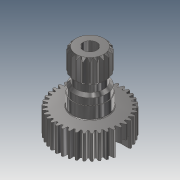
# Autodesk Inventor part: Цилиндрическое зубчатое зацепление2
Saved by Autodesk Inventor 2017 (Build 210142000, 142)
## iProperties
Created: 2018-08-24
Part Number: Цилиндрическое зубчатое зацепление2
Material: Сталь нержавеющая, 440C
Document SubType Name: Modeling
Designer: Shepelev
Categories: <?xml version="1.0" encoding="UTF-16"?> <MemberInstance><Categories><FamilyTemplate><FamilyTemplateParameter ValueType="xs:double" Id="1" ObjectReferenceKey="da_z" ObjectType="kUserParameterObject"/><FamilyTemplateParameter ValueType="xs:double" Id="2" ObjectReferenceKey="da_b" ObjectType="kUserParameterObject"/><FamilyTemplateParameter ValueType="xs:double" Id="3" ObjectReferenceKey="da_beta" ObjectType="kUserParameterObject"/><FamilyTemplateParameter ValueType="xs:double" Id="4" ObjectReferenceKey="da_da" ObjectType="kUserParameterObject"/><FamilyTemplateParameter ValueType="xs:double" Id="5" ObjectReferenceKey="da_aw" ObjectType="kUserParameterObject"/><FamilyTemplateParameter ValueType="xs:string" Id="6" ObjectReferenceKey="EAIAABAAAACIAQAAAAAAAIAAAAAAAAAA" ObjectType="83910656" SubObjectId="SurfaceGeometry"/></FamilyTemplate><ParamToTemplateMap><ParamToTemplate CategoryParameter="//CategoryParameter[@InternalName='046C89C9-8512-4d59-83FE-43B91F4F132A']" TemplateParameter="1"/><ParamToTemplate CategoryParameter="//CategoryParameter[@InternalName='2552DF32-E462-4b46-AEBF-C6C7768E72AC']" TemplateParameter="2"/><ParamToTemplate CategoryParameter="//CategoryParameter[@InternalName='C9EE641D-15FC-4fae-A226-E94C4372FDD7']" TemplateParameter="3"/><ParamToTemplate><ParamToTemplate CategoryParameter="//CategoryParameter[@InternalName='00B6519A-459B-49c7-AD84-2E56D39A5744']" ConstantValue="-0.270000"/></ParamToTemplate><ParamToTemplate><ParamToTemplate CategoryParameter="//CategoryParameter[@InternalName='04B31F0E-C7A6-4894-AA32-9629BEFACF47']" ConstantValue="1.000000"/></ParamToTemplate><ParamToTemplate><ParamToTemplate CategoryParameter="//CategoryParameter[@InternalName='43CBEC2E-7847-49e7-A936-2F7889FCB2D9']" ConstantValue="0.250000"/></ParamToTemplate><ParamToTemplate><ParamToTemplate CategoryParameter="//CategoryParameter[@InternalName='B1EFC894-105D-4ebd-86BF-FA20ED196853']" ConstantValue="0.350000"/></ParamToTemplate><ParamToTemplate><ParamToTemplate CategoryParameter="//CategoryParameter[@InternalName='51175063-3D10-4879-93E8-6246FE8B403D']" ConstantValue="2060000000.000000"/></ParamToTemplate><ParamToTemplate><ParamToTemplate CategoryParameter="//CategoryParameter[@InternalName='A3A52E27-4454-46a9-B0BD-C932399B70AF']" ConstantValue="0.300000"/></ParamToTemplate><ParamToTemplate><ParamToTemplate CategoryParameter="//CategoryParameter[@InternalName='91B76062-C214-41d9-B1B9-14D2AB99603D']" ConstantValue="0.025000"/></ParamToTemplate><ParamToTemplate><ParamToTemplate CategoryParameter="//CategoryParameter[@InternalName='374E806E-8B8A-4dda-A9AA-1039D6500AD2']" ConstantValue="40.000000"/></ParamToTemplate><ParamToTemplate><ParamToTemplate CategoryParameter="//CategoryParameter[@InternalName='2D373A89-B862-43d6-8D0B-0CBF12AB9F6C']" ConstantValue="0.349066"/></ParamToTemplate><ParamToTemplate CategoryParameter="//CategoryParameter[@InternalName='37777632-D6A2-4fac-9D53-DB8ACD95C989']" TemplateParameter="4"/><ParamToTemplate CategoryParameter="//CategoryParameter[@InternalName='FD1017F1-B727-4f7e-9707-0F86F1FF9423']" TemplateParameter="5"/><ParamToTemplate><ParamToTemplate CategoryParameter="//CategoryParameter[@InternalName='9E1B4470-B2D3-4ff1-B813-535BB4CDF51A']" ConstantValue="3520000.000000"/></ParamToTemplate><ParamToTemplate><ParamToTemplate CategoryParameter="//CategoryParameter[@InternalName='F8452263-BFF6-458c-9FB1-07C4B99E95CD']" ConstantValue="11400000.000000"/></ParamToTemplate><ParamToTemplate><ParamToTemplate CategoryParameter="//CategoryParameter[@InternalName='3E3BB259-FD49-497f-8171-6EBC954A3479']" ConstantValue="2.000000"/></ParamToTemplate><ParamToTemplate CategoryParameter="//CategoryParameter[@InternalName='27C3BAF2-7550-4e4b-AE2C-0DB134B7D9B7']" TemplateParameter="6"/></ParamToTemplateMap><Category DisplayName="Gear" InternalName="DC85795E-93AB-48d5-8EEE-5A27447B64BD" Mnemonic="Gear"><CategoryParameter DisplayName="z" InternalName="046C89C9-8512-4d59-83FE-43B91F4F132A" Mnemonic="z"/><CategoryParameter DisplayName="b" InternalName="2552DF32-E462-4b46-AEBF-C6C7768E72AC" Mnemonic="b"/><CategoryParameter DisplayName="||b|" InternalName="C9EE641D-15FC-4fae-A226-E94C4372FDD7" Mnemonic="beta"/><CategoryParameter DisplayName="x" InternalName="00B6519A-459B-49c7-AD84-2E56D39A5744" Mnemonic="x"/><CategoryParameter DisplayName="a*" InternalName="04B31F0E-C7A6-4894-AA32-9629BEFACF47" Mnemonic="a"/><CategoryParameter DisplayName="c*" InternalName="43CBEC2E-7847-49e7-A936-2F7889FCB2D9" Mnemonic="c"/><CategoryParameter DisplayName="r|.f|*" InternalName="B1EFC894-105D-4ebd-86BF-FA20ED196853" Mnemonic="rf"/><CategoryParameter DisplayName="E" InternalName="51175063-3D10-4879-93E8-6246FE8B403D" Mnemonic="E"/><CategoryParameter DisplayName="||m|" InternalName="A3A52E27-4454-46a9-B0BD-C932399B70AF" Mnemonic="mi"/><Category DisplayName="SpurGear" InternalName="26C5A22E-A91E-4dfd-A3B3-23CCAFAE1764" Mnemonic="SpurGear"><CategoryParameter DisplayName="m" InternalName="91B76062-C214-41d9-B1B9-14D2AB99603D" Mnemonic="m"/><CategoryParameter DisplayName="P" InternalName="374E806E-8B8A-4dda-A9AA-1039D6500AD2" Mnemonic="PP"/><CategoryParameter DisplayName="||a|" InternalName="2D373A89-B862-43d6-8D0B-0CBF12AB9F6C" Mnemonic="alpha"/><CategoryParameter DisplayName="d|.a|" InternalName="37777632-D6A2-4fac-9D53-DB8ACD95C989" Mnemonic="da"/><CategoryParameter DisplayName="a|.w|" InternalName="FD1017F1-B727-4f7e-9707-0F86F1FF9423" Mnemonic="aw"/><CategoryParameter DisplayName="||s||.Flim|" InternalName="9E1B4470-B2D3-4ff1-B813-535BB4CDF51A" Mnemonic="sFlim"/><CategoryParameter DisplayName="||s||.Hlim|" InternalName="F8452263-BFF6-458c-9FB1-07C4B99E95CD" Mnemonic="sHlim"/><CategoryParameter DisplayName="тип" InternalName="3E3BB259-FD49-497f-8171-6EBC954A3479" Mnemonic="type"/><CategoryParameter DisplayName="PitchDiameter" InternalName="27C3BAF2-7550-4e4b-AE2C-0DB134B7D9B7" Mnemonic="IDS_PITCHDIAM"/></Category></Category></Categories></MemberInstance>
Density: 7.75 g/cm^3
Appearance: С умеренной полировкой
CustomPartVersion: 1
Author: Shepelev
Autodesk Inventor part; units mm, degrees
ref_plane "YZ Plane" through (0, 0, 0) normal (1, 0, 0) x (0, 1, 0)
ref_plane "XZ Plane" through (0, 0, 0) normal (0, 1, 0) x (-1, 0, 0)
ref_plane "XY Plane" through (0, 0, 0) normal (0, 0, 1) x (1, 0, 0)
sketch "Sketch1" plane through (0, 0, 0) normal (0, 0, 1) x (1, 0, 0)
  circle A0 centre (0, 0) radius 4.9325
  dimension "d0" = 9.865
  constraints: 1 centre point
  measures "d0" diameter of A0
extrude "Extrusion1" add sketch "Sketch1" along normal blind 3.5
ref_plane "Work Plane2" through (0, 0, 1.75) normal (0, 0, 1) x (1, 0, 0)
sketch "Sketch2" plane through (0, 0, 0) normal (0, 0, -1) x (-1, 0, 0)
  circle A0 centre (0, 0) radius 4.9325 projected
  circle A1 centre (0, 0) radius 4.75
  dimension "d3" = 9.5
  constraints: 1 centre point, 1 coincident
  measures "d3" diameter of A1
surface extrude "Средний диаметр" sketch "Sketch2" against normal through all shown no curves A1
ref_plane "Work Plane8" through (0, 0, 0) normal (0.9965845, 0.0825793, 0) x (0, 0, 1)
ref_plane "Work Plane9" through (0, 0, 0) normal (1, 0, 0) x (0, 1, 0)
spur gear teeth "Цилиндрическое зубчатое зацепление" teeth 38 pitch diameter 9.5 tip diameter 9.865 root diameter 8.74 face width 3.5 start plane through (0, 0, 0) normal (0, 0, -1) x (-1, 0, 0)
sketch "Эскиз3" plane through (0, 0, 0) normal (1, 0, 0) x (0, 1, 0)
  line L0 (-6.9055, 0) -> (6.9055, 0) projected
  line L1 (0, -0.7) -> (0, 4.2) projected
  line L2 (0, 11) -> (2.4, 11)
  line L3 (2.4, 11) -> (2.4, 7.6)
  line L4 (2.4, 7.6) -> (2, 7.6)
  line L5 (2, 7.6) -> (2, 6.6)
  line L6 (2, 6.6) -> (2.4, 6.6)
  line L7 (2.4, 6.6) -> (2.4, 5.25)
  line L8 (2.4, 5.25) -> (2.5, 5.25)
  line L9 (2.5, 5.25) -> (2.5, 3.5)
  line L10 (2.5, 3.5) -> (0, 3.5)
  line L11 (0, 11) -> (0, 3.5)
  line L12 (-0.0903, 3.5) -> (-0.3056, 3.5) projected
  point P0 (0, 0)
  dimension "d49" = 7.5
  dimension "d50" = 4.8
  dimension "d51" = 4
  dimension "d52" = 4.8
  dimension "d53" = 5
  dimension "d55" = 1.75
  dimension "d56" = 1
  dimension "d57" = 4.1
  dimension "d58" = 3.4
  constraints: 20 end point, 5 perpendicular, 3 point on line, 2 collinear, 2 parallel, 1 horizontal
  measures "d49" distance of L2.start L10.end
  measures "d50" diameter of L3 L1
  measures "d51" diameter of L5 L1
  measures "d52" diameter of L7 L1
  measures "d53" diameter of L9 L1
  measures "d55" distance of L8.end L9.end
  measures "d56" distance of L4.end L5.end
  measures "d57" distance between parallel lines of L10 L4
  measures "d58" distance of L2.end L3.end
revolve "Вращение1" add sketch "Эскиз3" angle 360 about axis through (0, 0, 0) along (0, 0, 1)
fillet "Сопряжение1" radius 0.1 1 edges at (0, -2.5, 3.5)
chamfer "Фаска1" distance 0.4 angle 45 3 edges at (0, -2.4, 7.6) (0, -2.4, 11) (0, -2.4, 6.6)
sketch "Эскиз4" plane through (0, 0, 0) normal (0, 0, -1) x (-1, 0, 0)
  point P0 (0, 0)
hole "Отверстие1" at (0, 0, 0) direction (0, 0, 1) diameter 2.013 depth 11 tip angle 118 counterbore diameter 3.4 counterbore depth 4.5 thread size "M2.5" designation "M2,5" class "6H" standard "ISO Metric profile"
chamfer "Фаска2" distance 0.2 angle 45 1 edges at (0, -1.0065, 4.5)
sketch "Эскиз5" plane through (0, 0, 0) normal (0, 0, -1) x (-1, 0, 0)
  circle A0 centre (0, 0) radius 3.5
  dimension "d74" = 7
  constraints: 1 centre point, 1 coincident
  measures "d74" diameter of A0
extrude "Выдавливание2" cut sketch "Эскиз5" against normal blind 1
sketch "Эскиз6" plane through (0, 0, 0) normal (0, 0, -1) x (-1, 0, 0)
  line L0 (-6, 1) -> (0, 1)
  line L1 (0, 1) -> (0, -1)
  line L2 (0, -1) -> (-6, -1)
  line L3 (-6, -1) -> (-6, 1)
  point P0 (0, 0)
  point P1 (0, 0)
  dimension "d77" = 6
  dimension "d78" = 2
  constraints: 8 end point, 2 parallel, 1 coincident, 1 horizontal, 1 midpoint, 1 perpendicular
  measures "d77" distance of L0.start L0.end
  measures "d78" distance of L2.end L0.start
extrude "Выдавливание3" cut sketch "Эскиз6" against normal blind 1.5
sketch "Эскиз7" plane through (0, 0, 11) normal (0, 0, 1) x (1, 0, 0)
  circle A0 centre (0, 0) radius 2.4 projected
  circle A1 centre (0, 0) radius 2 projected
  circle A2 centre (0, 0) radius 2.4 projected
  circle A3 centre (0, 0) radius 2 projected
  line L0 (0.3754, 2.3705) -> (0, 0) construction
  line L1 (0, 0) -> (-0.3754, 2.3705) construction
  line L2 (0, -6.9055) -> (0, 6.9055) projected
  line L3 (-6.8922, 0) -> (6.8922, 0) projected
  arc A4 (-0.326, 2.3778) -> (-0.3754, 2.3705) centre (0, 0) ccw
  arc A5 (0.3754, 2.3705) -> (0.326, 2.3778) centre (0, 0) ccw
  arc A6 (0.05, 1.9994) -> (-0.05, 1.9994) centre (0, 0) ccw
  line L4 (-0.326, 2.3778) -> (-0.05, 1.9994)
  line L5 (0.05, 1.9994) -> (0.326, 2.3778)
  arc A7 (0.326, 2.3778) -> (-0.326, 2.3778) centre (0, 0) ccw
  point P0 (0, 2)
  dimension "d82" = 18
  dimension "d86" = 0.05
  dimension "d87" = 0.05
  dimension "d88" = 0.1
  constraints: 21 point on circle, 8 end point, 4 centre point, 4 concentric, 1 point on line, 1 other
  measures "d82" angle of L0 L1
  measures "d86" distance from line of L1 L4.start
  measures "d87" distance from line of L5.end L0
  measures "d88" distance of L5.start L4.end
extrude "Выдавливание4" cut sketch "Эскиз7" against normal blind 3.5 contours L5 A1 L2 A0 | L2 A1 L4 A0
pattern_circular "Круговой массив1" count 20 over 360 about axis through (0, 0, 9.3) along (0, 0, -1) of "Выдавливание4"
equation "\"d0\" = da_da"
equation "\"d1\" = da_b"
equation "\"d3\" = da_dw"
equation "\"d16\" = da_aw"
equation "\"d43\" = da_aw"
equation "\"d46\" = da_aw"
equation "\"da_da\" = 9.865"
equation "\"da_b\" = 3.5"
equation "\"da_dw\" = 9.5"
equation "\"da_aw\" = 6"
body "Solid1"
body "Srf1"
